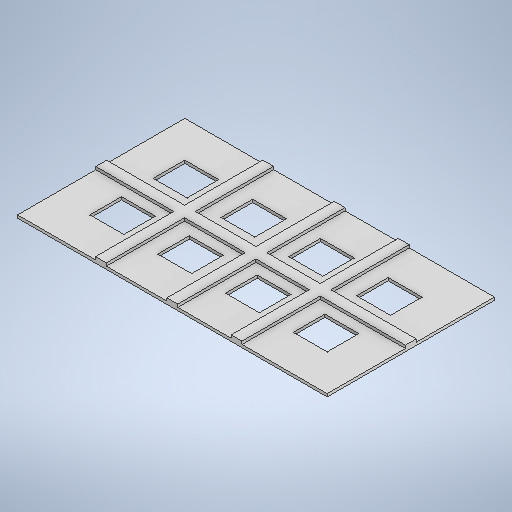
# Autodesk Inventor part: test_front_cover
Saved by Autodesk Inventor 2025 (Build 290162000, 162)
## iProperties
Created: 2025-05-08
Part Number: test_front_cover
Material: Generic
Document SubType Name: Modeling
Designer: ethan
Density: 1 g/cm^3
Appearance: Default
Author: ethan
Autodesk Inventor part; units mm, degrees
ref_plane "YZ Plane" through (0, 0, 0) normal (1, 0, 0) x (0, 1, 0)
ref_plane "XZ Plane" through (0, 0, 0) normal (0, 1, 0) x (-1, 0, 0)
ref_plane "XY Plane" through (0, 0, 0) normal (0, 0, 1) x (1, 0, 0)
sketch "Sketch1" plane through (0, 0, 0) normal (0, 1, 0) x (-1, 0, 0)
  line L0 (0, 0) -> (-25.4, 0) construction
  line L1 (-25.4, 0) -> (-25.4, -25.4) construction
  line L2 (-25.4, -25.4) -> (0, -25.4) construction
  line L3 (0, -25.4) -> (0, 0) construction
  line L4 (-25.4, -25.4) -> (-49.2125, -25.4) construction
  line L5 (-49.2125, -25.4) -> (-49.2125, -47.625) construction
  line L6 (-49.2125, -47.625) -> (-25.4, -47.625) construction
  line L7 (-25.4, -47.625) -> (-25.4, -25.4) construction
  line L8 (-73.025, -25.4) -> (-96.8375, -25.4) construction
  line L9 (-96.8375, -25.4) -> (-96.8375, -47.625) construction
  line L10 (-96.8375, -47.625) -> (-73.025, -47.625) construction
  line L11 (-73.025, -47.625) -> (-73.025, -25.4) construction
  line L12 (-120.65, -25.4) -> (-144.4625, -25.4) construction
  line L13 (-144.4625, -25.4) -> (-144.4625, -47.625) construction
  line L14 (-144.4625, -47.625) -> (-120.65, -47.625) construction
  line L15 (-120.65, -47.625) -> (-120.65, -25.4) construction
  line L16 (-168.275, -25.4) -> (-192.0875, -25.4) construction
  line L17 (-192.0875, -25.4) -> (-192.0875, -47.625) construction
  line L18 (-192.0875, -47.625) -> (-168.275, -47.625) construction
  line L19 (-168.275, -47.625) -> (-168.275, -25.4) construction
  line L20 (-25.4, -69.85) -> (-49.2125, -69.85) construction
  line L21 (-49.2125, -69.85) -> (-49.2125, -92.075) construction
  line L22 (-49.2125, -92.075) -> (-25.4, -92.075) construction
  line L23 (-25.4, -92.075) -> (-25.4, -69.85) construction
  line L24 (-73.025, -69.85) -> (-96.8375, -69.85) construction
  line L25 (-96.8375, -69.85) -> (-96.8375, -92.075) construction
  line L26 (-96.8375, -92.075) -> (-73.025, -92.075) construction
  line L27 (-73.025, -92.075) -> (-73.025, -69.85) construction
  line L28 (-120.65, -69.85) -> (-144.4625, -69.85) construction
  line L29 (-144.4625, -69.85) -> (-144.4625, -92.075) construction
  line L30 (-144.4625, -92.075) -> (-120.65, -92.075) construction
  line L31 (-120.65, -92.075) -> (-120.65, -69.85) construction
  line L32 (-168.275, -69.85) -> (-192.0875, -69.85) construction
  line L33 (-192.0875, -69.85) -> (-192.0875, -92.075) construction
  line L34 (-192.0875, -92.075) -> (-168.275, -92.075) construction
  line L35 (-168.275, -92.075) -> (-168.275, -69.85) construction
  line L36 (-192.0875, -92.075) -> (-217.4875, -92.075) construction
  line L37 (-217.4875, -92.075) -> (-217.4875, -117.475) construction
  line L38 (-217.4875, -117.475) -> (-192.0875, -117.475) construction
  line L39 (-192.0875, -117.475) -> (-192.0875, -92.075) construction
  line L40 (0, 0) -> (-217.4875, 0)
  line L41 (-217.4875, 0) -> (-217.4875, -117.475)
  line L42 (-217.4875, -117.475) -> (0, -117.475)
  line L43 (0, -117.475) -> (0, 0)
  line L44 (-192.0875, -92.075) -> (-168.275, -92.075)
  line L45 (-168.275, -92.075) -> (-168.275, -69.85)
  line L46 (-168.275, -69.85) -> (-192.0875, -69.85)
  line L47 (-192.0875, -69.85) -> (-192.0875, -92.075)
  line L48 (-144.4625, -92.075) -> (-120.65, -92.075)
  line L49 (-120.65, -92.075) -> (-120.65, -69.85)
  line L50 (-120.65, -69.85) -> (-144.4625, -69.85)
  line L51 (-144.4625, -69.85) -> (-144.4625, -92.075)
  line L52 (-96.8375, -92.075) -> (-73.025, -92.075)
  line L53 (-73.025, -92.075) -> (-73.025, -69.85)
  line L54 (-73.025, -69.85) -> (-96.8375, -69.85)
  line L55 (-96.8375, -69.85) -> (-96.8375, -92.075)
  line L56 (-49.2125, -92.075) -> (-25.4, -92.075)
  line L57 (-25.4, -92.075) -> (-25.4, -69.85)
  line L58 (-25.4, -69.85) -> (-49.2125, -69.85)
  line L59 (-49.2125, -69.85) -> (-49.2125, -92.075)
  line L60 (-25.4, -47.625) -> (-49.2125, -47.625)
  line L61 (-49.2125, -47.625) -> (-49.2125, -25.4)
  line L62 (-49.2125, -25.4) -> (-25.4, -25.4)
  line L63 (-25.4, -25.4) -> (-25.4, -47.625)
  line L64 (-73.025, -47.625) -> (-96.8375, -47.625)
  line L65 (-96.8375, -47.625) -> (-96.8375, -25.4)
  line L66 (-96.8375, -25.4) -> (-73.025, -25.4)
  line L67 (-73.025, -25.4) -> (-73.025, -47.625)
  line L68 (-120.65, -47.625) -> (-144.4625, -47.625)
  line L69 (-144.4625, -47.625) -> (-144.4625, -25.4)
  line L70 (-144.4625, -25.4) -> (-120.65, -25.4)
  line L71 (-120.65, -25.4) -> (-120.65, -47.625)
  line L72 (-168.275, -47.625) -> (-192.0875, -47.625)
  line L73 (-192.0875, -47.625) -> (-192.0875, -25.4)
  line L74 (-192.0875, -25.4) -> (-168.275, -25.4)
  line L75 (-168.275, -25.4) -> (-168.275, -47.625)
  dimension "d1" = 25.4
  dimension "d2" = 23.8125
  dimension "d3" = 22.225
  dimension "d6" = 47.625
  dimension "d9" = 44.45
  dimension "d12" = 25.4
  dimension "d13" = 25.4
  constraints: 152 end point, 24 parallel, 13 horizontal, 12 perpendicular, 2 collinear, 1 vertical, 54 other
  measures "d1" distance of L1.end L0.end
  measures "d2" distance of L6.end L5.end
  measures "d3" distance of L5.end L4.end
  measures "d6" distance of L1.end L8.start
  measures "d9" distance of L1.end L20.start
  measures "d12" distance of L38.end L37.end
  measures "d13" distance of L37.end L36.end
extrude "Extrusion1" add sketch "Sketch1" along normal blind 2
sketch "Sketch2" plane through (0, 2, 0) normal (0, 1, 0) x (1, 0, 0)
  line L0 (217.4875, 0) -> (217.4875, 117.475) construction
  line L1 (217.4875, 117.475) -> (0, 117.475) construction
  line L2 (0, 117.475) -> (0, 0) construction
  line L3 (0, 0) -> (217.4875, 0) construction
  line L4 (168.275, 47.625) -> (192.0875, 47.625) construction
  line L5 (192.0875, 47.625) -> (192.0875, 25.4) construction
  line L6 (192.0875, 25.4) -> (168.275, 25.4) construction
  line L7 (168.275, 25.4) -> (168.275, 47.625) construction
  line L8 (120.65, 47.625) -> (144.4625, 47.625) construction
  line L9 (144.4625, 47.625) -> (144.4625, 25.4) construction
  line L10 (144.4625, 25.4) -> (120.65, 25.4) construction
  line L11 (120.65, 25.4) -> (120.65, 47.625) construction
  line L12 (73.025, 47.625) -> (96.8375, 47.625) construction
  line L13 (96.8375, 47.625) -> (96.8375, 25.4) construction
  line L14 (96.8375, 25.4) -> (73.025, 25.4) construction
  line L15 (73.025, 25.4) -> (73.025, 47.625) construction
  line L16 (25.4, 47.625) -> (49.2125, 47.625) construction
  line L17 (49.2125, 47.625) -> (49.2125, 25.4) construction
  line L18 (49.2125, 25.4) -> (25.4, 25.4) construction
  line L19 (25.4, 25.4) -> (25.4, 47.625) construction
  line L20 (49.2125, 92.075) -> (49.2125, 69.85) construction
  line L21 (49.2125, 69.85) -> (25.4, 69.85) construction
  line L22 (25.4, 69.85) -> (25.4, 92.075) construction
  line L23 (25.4, 92.075) -> (49.2125, 92.075) construction
  line L24 (96.8375, 92.075) -> (96.8375, 69.85) construction
  line L25 (96.8375, 69.85) -> (73.025, 69.85) construction
  line L26 (73.025, 69.85) -> (73.025, 92.075) construction
  line L27 (73.025, 92.075) -> (96.8375, 92.075) construction
  line L28 (144.4625, 92.075) -> (144.4625, 69.85) construction
  line L29 (144.4625, 69.85) -> (120.65, 69.85) construction
  line L30 (120.65, 69.85) -> (120.65, 92.075) construction
  line L31 (120.65, 92.075) -> (144.4625, 92.075) construction
  line L32 (192.0875, 92.075) -> (192.0875, 69.85) construction
  line L33 (192.0875, 69.85) -> (168.275, 69.85) construction
  line L34 (168.275, 69.85) -> (168.275, 92.075) construction
  line L35 (168.275, 92.075) -> (192.0875, 92.075) construction
  line L36 (0, 54.9275) -> (217.4875, 54.9275) construction
  line L37 (217.4875, 54.9275) -> (217.4875, 62.5475) construction
  line L38 (217.4875, 62.5475) -> (0, 62.5475) construction
  line L39 (0, 62.5475) -> (0, 54.9275) construction
  line L40 (0, 54.9275) -> (217.4875, 62.5475) construction
  line L41 (217.4875, 54.9275) -> (0, 62.5475) construction
  line L42 (104.9338, 0) -> (112.5538, 0) construction
  line L43 (112.5538, 0) -> (112.5537, 117.475) construction
  line L44 (112.5537, 117.475) -> (104.9337, 117.475) construction
  line L45 (104.9337, 117.475) -> (104.9338, 0) construction
  line L46 (104.9338, 0) -> (112.5537, 117.475) construction
  line L47 (112.5538, 0) -> (104.9337, 117.475) construction
  line L48 (0, 62.5475) -> (217.4875, 62.5475)
  line L49 (217.4875, 62.5475) -> (217.4875, 54.9275)
  line L50 (217.4875, 54.9275) -> (0, 54.9275)
  line L51 (0, 54.9275) -> (0, 62.5475)
  line L52 (104.9337, 117.475) -> (112.5537, 117.475)
  line L53 (112.5537, 117.475) -> (112.5538, 0)
  line L54 (112.5538, 0) -> (104.9338, 0)
  line L55 (104.9338, 0) -> (104.9337, 117.475)
  line L56 (49.2125, 92.075) -> (73.025, 92.075) construction
  line L57 (73.025, 92.075) -> (73.025, 69.85) construction
  line L58 (73.025, 69.85) -> (49.2125, 69.85) construction
  line L59 (49.2125, 69.85) -> (49.2125, 92.075) construction
  line L60 (168.275, 92.075) -> (144.4625, 92.075) construction
  line L61 (144.4625, 92.075) -> (144.4625, 69.85) construction
  line L62 (144.4625, 69.85) -> (168.275, 69.85) construction
  line L63 (168.275, 69.85) -> (168.275, 92.075) construction
  line L64 (217.4875, 117.475) -> (0, 117.475) projected
  line L65 (54.7688, 0) -> (62.3888, 0)
  line L66 (62.3888, 0) -> (62.3888, 117.475)
  line L67 (62.3888, 117.475) -> (54.7688, 117.475)
  line L68 (54.7688, 117.475) -> (54.7688, 0)
  line L69 (54.7688, 0) -> (62.3888, 117.475) construction
  line L70 (62.3888, 0) -> (54.7688, 117.475) construction
  line L71 (150.0187, 0) -> (157.6388, 0)
  line L72 (157.6388, 0) -> (157.6387, 117.475)
  line L73 (157.6387, 117.475) -> (150.0187, 117.475)
  line L74 (150.0187, 117.475) -> (150.0187, 0)
  line L75 (150.0187, 0) -> (157.6387, 117.475) construction
  line L76 (157.6388, 0) -> (150.0187, 117.475) construction
  point P0 (108.7438, 58.7375)
  point P1 (108.7438, 58.7375)
  point P2 (58.5787, 58.7375)
  point P3 (153.8288, 58.7375)
  point P4 (54.7688, 54.9275)
  point P5 (62.3888, 54.9275)
  point P6 (104.9338, 54.9275)
  point P7 (112.5538, 54.9275)
  point P8 (150.0187, 54.9275)
  point P9 (157.6388, 54.9275)
  point P10 (157.6388, 62.5475)
  point P11 (150.0187, 62.5475)
  point P12 (112.5537, 62.5475)
  point P13 (104.9338, 62.5475)
  point P14 (62.3888, 62.5475)
  point P15 (54.7688, 62.5475)
  dimension "d16" = 7.62
  dimension "d17" = 7.62
  dimension "d18" = 7.62
  dimension "d19" = 7.62
  constraints: 80 end point, 16 parallel, 9 midpoint, 8 horizontal, 8 perpendicular, 4 point on line
  measures "d16" distance of L37.end L36.end
  measures "d17" distance of L44.end L43.end
  measures "d18" distance of L67.end L66.end
  measures "d19" distance of L73.end L72.end
extrude "Extrusion2" add sketch "Sketch2" along normal blind 2 contours L48 L68 L50 L51 | L68 L64 L66 L48 | L48 L66 L50 L68 | L48 L55 L50 L66 | L50 L66 L65 L68 | L55 L52 L53 L48 | L48 L53 L50 L55 | L48 L74 L50 L53 | L50 L53 L54 L55 | L74 L64 L72 L48 | L48 L72 L50 L74 | L48 L49 L50 L72 | L50 L72 L71 L74
body "Solid1"
